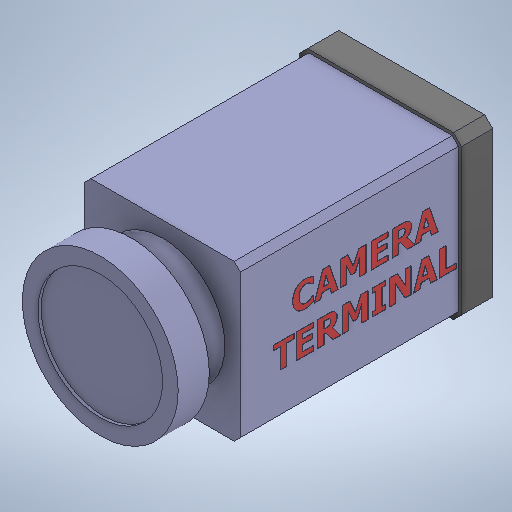
# Autodesk Inventor part: CAMERA TERMINAL
Saved by Autodesk Inventor 2025 (Build 290162000, 162)
## iProperties
Created: 2024-09-26
Part Number: CAMERA TERMINAL
Material: Generic
Document SubType Name: Modeling
Designer: DMIADX
Density: 1 g/cm^3
Appearance: Slate Blue
Author: DMIADX
Autodesk Inventor part; units mm, degrees
ref_plane "YZ Plane" through (0, 0, 0) normal (1, 0, 0) x (0, 1, 0)
ref_plane "XZ Plane" through (0, 0, 0) normal (0, 1, 0) x (-1, 0, 0)
ref_plane "XY Plane" through (0, 0, 0) normal (0, 0, 1) x (1, 0, 0)
sketch "Sketch1" plane through (0, 0, 0) normal (0, 0, 1) x (1, 0, 0)
  line L0 (25, -25) -> (-25, -25)
  line L1 (-25, -25) -> (-25, 25)
  line L2 (-25, 25) -> (25, 25)
  line L3 (25, 25) -> (25, -25)
  line L4 (25, -25) -> (-25, 25) construction
  line L5 (-25, -25) -> (25, 25) construction
  point P0 (0, 0)
  dimension "d0" = 50
  dimension "d1" = 50
  constraints: 12 end point, 2 midpoint, 2 parallel, 1 horizontal, 1 perpendicular
  measures "d0" distance of L1.end L2.end
  measures "d1" distance of L0.end L1.end
extrude "Extrusion1" add sketch "Sketch1" along normal blind 80
sketch "Sketch2" plane through (0, 0, 80) normal (0, 0, 1) x (1, 0, 0)
  circle A0 centre (0, 0) radius 25
  circle A1 centre (0, 0) radius 20
  dimension "d4" = 50
  dimension "d5" = 40
  constraints: 2 centre point, 2 coincident
  measures "d4" diameter of A0
  measures "d5" diameter of A1
extrude "Extrusion2" add sketch "Sketch2" along normal blind 19 contours A1
extrude "Extrusion3" add sketch "Sketch2" along normal blind 20
extrude "Extrusion4" cut sketch "Sketch2" along normal blind 10
sketch "Sketch3" plane through (25, -25, 0) normal (1, 0, 0) x (0, 0, -1)
  line L0 (-80, 50) -> (0, 50) construction
  line L1 (0, 50) -> (0, 0) construction
  line L2 (0, 0) -> (-80, 0) construction
  line L3 (-80, 0) -> (-80, 50) construction
  spline S0 degree 2 poles (-59.2512, 27.3525) (-61.0535, 27.3525) (-63.1669, 29.5308) (-63.1669, 31.5016) knots 0 0 0 1 2 2 2
  spline S1 degree 2 poles (-63.1669, 31.5016) (-63.1669, 33.4011) (-61.047, 35.6637) (-59.2447, 35.6637) knots 0 0 0 1 2 2 2
  spline S2 degree 2 poles (-59.2447, 35.6637) (-58.7715, 35.6637) (-58.0065, 35.5535) (-57.6564, 35.4627) knots 0 0 0 1 2 2 2
  spline S3 degree 2 poles (-57.6564, 35.4627) (-57.3841, 35.3784) (-56.7423, 35.0997) (-56.5413, 34.9959) knots 0 0 0 1 2 2 2
  line L4 (-56.5413, 34.9959) -> (-56.5413, 33.0899)
  line L5 (-56.5413, 33.0899) -> (-56.7423, 33.0899)
  spline S4 degree 2 poles (-56.7423, 33.0899) (-56.8914, 33.2196) (-57.3323, 33.5827) (-57.611, 33.7512) knots 0 0 0 1 2 2 2
  spline S5 degree 2 poles (-57.611, 33.7512) (-57.8898, 33.9263) (-58.5575, 34.1661) (-58.9271, 34.1661) knots 0 0 0 1 2 2 2
  spline S6 degree 2 poles (-58.9271, 34.1661) (-59.3614, 34.1661) (-60.081, 33.8938) (-60.4117, 33.5502) knots 0 0 0 1 2 2 2
  spline S7 degree 2 poles (-60.4117, 33.5502) (-60.7099, 33.2455) (-61.0924, 32.2018) (-61.0924, 31.4951) knots 0 0 0 1 2 2 2
  spline S8 degree 2 poles (-61.0924, 31.4951) (-61.0924, 30.7496) (-60.6969, 29.7318) (-60.3728, 29.4206) knots 0 0 0 1 2 2 2
  spline S9 degree 2 poles (-60.3728, 29.4206) (-60.0616, 29.1159) (-59.2966, 28.8501) (-58.9141, 28.8501) knots 0 0 0 1 2 2 2
  spline S10 degree 2 poles (-58.9141, 28.8501) (-58.5186, 28.8501) (-57.799, 29.1159) (-57.5527, 29.278) knots 0 0 0 1 2 2 2
  spline S11 degree 2 poles (-57.5527, 29.278) (-57.2804, 29.44) (-56.872, 29.7836) (-56.7229, 29.9198) knots 0 0 0 1 2 2 2
  line L6 (-56.7229, 29.9198) -> (-56.5413, 29.9198)
  line L7 (-56.5413, 29.9198) -> (-56.5413, 28.0397)
  spline S12 degree 2 poles (-56.5413, 28.0397) (-56.7618, 27.936) (-57.3387, 27.6767) (-57.6499, 27.5859) knots 0 0 0 1 2 2 2
  spline S13 degree 2 poles (-57.6499, 27.5859) (-58.0259, 27.4692) (-58.6807, 27.3525) (-59.2512, 27.3525) knots 0 0 0 1 2 2 2
  line L8 (-56.2172, 27.5081) -> (-53.5138, 35.5081)
  line L9 (-53.5138, 35.5081) -> (-51.3225, 35.5081)
  line L10 (-51.3225, 35.5081) -> (-48.6191, 27.5081)
  line L11 (-48.6191, 27.5081) -> (-50.6872, 27.5081)
  line L12 (-50.6872, 27.5081) -> (-51.1864, 29.1418)
  line L13 (-51.1864, 29.1418) -> (-53.7018, 29.1418)
  line L14 (-53.7018, 29.1418) -> (-54.2075, 27.5081)
  line L15 (-54.2075, 27.5081) -> (-56.2172, 27.5081)
  line L16 (-51.6272, 30.594) -> (-52.4441, 33.2391)
  line L17 (-52.4441, 33.2391) -> (-53.2674, 30.594)
  line L18 (-53.2674, 30.594) -> (-51.6272, 30.594)
  line L19 (-39.6532, 27.5081) -> (-41.6499, 27.5081)
  line L20 (-41.6499, 27.5081) -> (-41.6499, 32.8112)
  line L21 (-41.6499, 32.8112) -> (-43.1021, 29.3882)
  line L22 (-43.1021, 29.3882) -> (-44.4765, 29.3882)
  line L23 (-44.4765, 29.3882) -> (-45.9287, 32.8112)
  line L24 (-45.9287, 32.8112) -> (-45.9287, 27.5081)
  line L25 (-45.9287, 27.5081) -> (-47.8217, 27.5081)
  line L26 (-47.8217, 27.5081) -> (-47.8217, 35.5081)
  line L27 (-47.8217, 35.5081) -> (-45.5073, 35.5081)
  line L28 (-45.5073, 35.5081) -> (-43.731, 31.56)
  line L29 (-43.731, 31.56) -> (-41.9676, 35.5081)
  line L30 (-41.9676, 35.5081) -> (-39.6532, 35.5081)
  line L31 (-39.6532, 35.5081) -> (-39.6532, 27.5081)
  line L32 (-37.9935, 27.5081) -> (-37.9935, 35.5081)
  line L33 (-37.9935, 35.5081) -> (-32.5867, 35.5081)
  line L34 (-32.5867, 35.5081) -> (-32.5867, 33.9846)
  line L35 (-32.5867, 33.9846) -> (-35.9968, 33.9846)
  line L36 (-35.9968, 33.9846) -> (-35.9968, 32.5778)
  line L37 (-35.9968, 32.5778) -> (-32.8525, 32.5778)
  line L38 (-32.8525, 32.5778) -> (-32.8525, 31.0543)
  line L39 (-32.8525, 31.0543) -> (-35.9968, 31.0543)
  line L40 (-35.9968, 31.0543) -> (-35.9968, 29.0316)
  line L41 (-35.9968, 29.0316) -> (-32.5867, 29.0316)
  line L42 (-32.5867, 29.0316) -> (-32.5867, 27.5081)
  line L43 (-32.5867, 27.5081) -> (-37.9935, 27.5081)
  line L44 (-23.8347, 27.5081) -> (-26.2788, 27.5081)
  line L45 (-26.2788, 27.5081) -> (-28.5024, 30.4449)
  line L46 (-28.5024, 30.4449) -> (-29.2285, 30.4449)
  line L47 (-29.2285, 30.4449) -> (-29.2285, 27.5081)
  line L48 (-29.2285, 27.5081) -> (-31.2253, 27.5081)
  line L49 (-31.2253, 27.5081) -> (-31.2253, 35.5081)
  line L50 (-31.2253, 35.5081) -> (-28.0097, 35.5081)
  spline S14 degree 2 poles (-28.0097, 35.5081) (-27.342, 35.5081) (-26.3566, 35.3395) (-25.9352, 35.0802) knots 0 0 0 1 2 2 2
  spline S15 degree 2 poles (-25.9352, 35.0802) (-25.5073, 34.8079) (-25.0016, 33.9587) (-25.0016, 33.3104) knots 0 0 0 1 2 2 2
  spline S16 degree 2 poles (-25.0016, 33.3104) (-25.0016, 32.3963) (-25.8314, 31.2488) (-26.5251, 30.9117) knots 0 0 0 1 2 2 2
  line L51 (-26.5251, 30.9117) -> (-23.8347, 27.5081)
  spline S17 degree 2 poles (-27.0632, 33.0575) (-27.0632, 33.3622) (-27.2966, 33.7966) (-27.5624, 33.9133) knots 0 0 0 1 2 2 2
  spline S18 degree 2 poles (-27.5624, 33.9133) (-27.7504, 33.9911) (-28.2107, 34.0365) (-28.5543, 34.0365) knots 0 0 0 1 2 2 2
  line L52 (-28.5543, 34.0365) -> (-29.2285, 34.0365)
  line L53 (-29.2285, 34.0365) -> (-29.2285, 31.8841)
  line L54 (-29.2285, 31.8841) -> (-28.6515, 31.8841)
  spline S19 degree 2 poles (-28.6515, 31.8841) (-28.2366, 31.8841) (-27.6467, 31.9878) (-27.4457, 32.1499) knots 0 0 0 1 2 2 2
  spline S20 degree 2 poles (-27.4457, 32.1499) (-27.2512, 32.3055) (-27.0632, 32.7204) (-27.0632, 33.0575) knots 0 0 0 1 2 2 2
  line L55 (-24.1005, 27.5081) -> (-21.3971, 35.5081)
  line L56 (-21.3971, 35.5081) -> (-19.2058, 35.5081)
  line L57 (-19.2058, 35.5081) -> (-16.5024, 27.5081)
  line L58 (-16.5024, 27.5081) -> (-18.5705, 27.5081)
  line L59 (-18.5705, 27.5081) -> (-19.0697, 29.1418)
  line L60 (-19.0697, 29.1418) -> (-21.5851, 29.1418)
  line L61 (-21.5851, 29.1418) -> (-22.0908, 27.5081)
  line L62 (-22.0908, 27.5081) -> (-24.1005, 27.5081)
  line L63 (-19.5105, 30.594) -> (-20.3274, 33.2391)
  line L64 (-20.3274, 33.2391) -> (-21.1507, 30.594)
  line L65 (-21.1507, 30.594) -> (-19.5105, 30.594)
  line L66 (-67.1053, 14.3363) -> (-67.1053, 20.8128)
  line L67 (-67.1053, 20.8128) -> (-69.4716, 20.8128)
  line L68 (-69.4716, 20.8128) -> (-69.4716, 22.3363)
  line L69 (-69.4716, 22.3363) -> (-62.7293, 22.3363)
  line L70 (-62.7293, 22.3363) -> (-62.7293, 20.8128)
  line L71 (-62.7293, 20.8128) -> (-65.0956, 20.8128)
  line L72 (-65.0956, 20.8128) -> (-65.0956, 14.3363)
  line L73 (-65.0956, 14.3363) -> (-67.1053, 14.3363)
  line L74 (-61.906, 14.3363) -> (-61.906, 22.3363)
  line L75 (-61.906, 22.3363) -> (-56.4992, 22.3363)
  line L76 (-56.4992, 22.3363) -> (-56.4992, 20.8128)
  line L77 (-56.4992, 20.8128) -> (-59.9092, 20.8128)
  line L78 (-59.9092, 20.8128) -> (-59.9092, 19.406)
  line L79 (-59.9092, 19.406) -> (-56.765, 19.406)
  line L80 (-56.765, 19.406) -> (-56.765, 17.8825)
  line L81 (-56.765, 17.8825) -> (-59.9092, 17.8825)
  line L82 (-59.9092, 17.8825) -> (-59.9092, 15.8598)
  line L83 (-59.9092, 15.8598) -> (-56.4992, 15.8598)
  line L84 (-56.4992, 15.8598) -> (-56.4992, 14.3363)
  line L85 (-56.4992, 14.3363) -> (-61.906, 14.3363)
  line L86 (-47.7472, 14.3363) -> (-50.1912, 14.3363)
  line L87 (-50.1912, 14.3363) -> (-52.4149, 17.2731)
  line L88 (-52.4149, 17.2731) -> (-53.141, 17.2731)
  line L89 (-53.141, 17.2731) -> (-53.141, 14.3363)
  line L90 (-53.141, 14.3363) -> (-55.1378, 14.3363)
  line L91 (-55.1378, 14.3363) -> (-55.1378, 22.3363)
  line L92 (-55.1378, 22.3363) -> (-51.9222, 22.3363)
  spline S21 degree 2 poles (-51.9222, 22.3363) (-51.2545, 22.3363) (-50.269, 22.1678) (-49.8477, 21.9084) knots 0 0 0 1 2 2 2
  spline S22 degree 2 poles (-49.8477, 21.9084) (-49.4198, 21.6361) (-48.9141, 20.7869) (-48.9141, 20.1386) knots 0 0 0 1 2 2 2
  spline S23 degree 2 poles (-48.9141, 20.1386) (-48.9141, 19.2245) (-49.7439, 18.077) (-50.4376, 17.7399) knots 0 0 0 1 2 2 2
  line L93 (-50.4376, 17.7399) -> (-47.7472, 14.3363)
  spline S24 degree 2 poles (-50.9757, 19.8857) (-50.9757, 20.1904) (-51.2091, 20.6248) (-51.4749, 20.7415) knots 0 0 0 1 2 2 2
  spline S25 degree 2 poles (-51.4749, 20.7415) (-51.6629, 20.8193) (-52.1232, 20.8647) (-52.4668, 20.8647) knots 0 0 0 1 2 2 2
  line L94 (-52.4668, 20.8647) -> (-53.141, 20.8647)
  line L95 (-53.141, 20.8647) -> (-53.141, 18.7123)
  line L96 (-53.141, 18.7123) -> (-52.564, 18.7123)
  spline S26 degree 2 poles (-52.564, 18.7123) (-52.1491, 18.7123) (-51.5592, 18.8161) (-51.3582, 18.9781) knots 0 0 0 1 2 2 2
  spline S27 degree 2 poles (-51.3582, 18.9781) (-51.1637, 19.1337) (-50.9757, 19.5486) (-50.9757, 19.8857) knots 0 0 0 1 2 2 2
  line L97 (-38.9822, 14.3363) -> (-40.9789, 14.3363)
  line L98 (-40.9789, 14.3363) -> (-40.9789, 19.6394)
  line L99 (-40.9789, 19.6394) -> (-42.4311, 16.2164)
  line L100 (-42.4311, 16.2164) -> (-43.8055, 16.2164)
  line L101 (-43.8055, 16.2164) -> (-45.2577, 19.6394)
  line L102 (-45.2577, 19.6394) -> (-45.2577, 14.3363)
  line L103 (-45.2577, 14.3363) -> (-47.1507, 14.3363)
  line L104 (-47.1507, 14.3363) -> (-47.1507, 22.3363)
  line L105 (-47.1507, 22.3363) -> (-44.8363, 22.3363)
  line L106 (-44.8363, 22.3363) -> (-43.06, 18.3882)
  line L107 (-43.06, 18.3882) -> (-41.2966, 22.3363)
  line L108 (-41.2966, 22.3363) -> (-38.9822, 22.3363)
  line L109 (-38.9822, 22.3363) -> (-38.9822, 14.3363)
  line L110 (-33.342, 14.3363) -> (-37.6467, 14.3363)
  line L111 (-37.6467, 14.3363) -> (-37.6467, 15.7302)
  line L112 (-37.6467, 15.7302) -> (-36.4992, 15.7302)
  line L113 (-36.4992, 15.7302) -> (-36.4992, 20.9425)
  line L114 (-36.4992, 20.9425) -> (-37.6467, 20.9425)
  line L115 (-37.6467, 20.9425) -> (-37.6467, 22.3363)
  line L116 (-37.6467, 22.3363) -> (-33.342, 22.3363)
  line L117 (-33.342, 22.3363) -> (-33.342, 20.9425)
  line L118 (-33.342, 20.9425) -> (-34.4895, 20.9425)
  line L119 (-34.4895, 20.9425) -> (-34.4895, 15.7302)
  line L120 (-34.4895, 15.7302) -> (-33.342, 15.7302)
  line L121 (-33.342, 15.7302) -> (-33.342, 14.3363)
  line L122 (-25.154, 14.3363) -> (-27.0859, 14.3363)
  line L123 (-27.0859, 14.3363) -> (-30.1718, 19.9117)
  line L124 (-30.1718, 19.9117) -> (-30.1718, 14.3363)
  line L125 (-30.1718, 14.3363) -> (-32.0065, 14.3363)
  line L126 (-32.0065, 14.3363) -> (-32.0065, 22.3363)
  line L127 (-32.0065, 22.3363) -> (-29.543, 22.3363)
  line L128 (-29.543, 22.3363) -> (-26.9887, 17.7528)
  line L129 (-26.9887, 17.7528) -> (-26.9887, 22.3363)
  line L130 (-26.9887, 22.3363) -> (-25.154, 22.3363)
  line L131 (-25.154, 22.3363) -> (-25.154, 14.3363)
  line L132 (-24.389, 14.3363) -> (-21.6856, 22.3363)
  line L133 (-21.6856, 22.3363) -> (-19.4943, 22.3363)
  line L134 (-19.4943, 22.3363) -> (-16.7909, 14.3363)
  line L135 (-16.7909, 14.3363) -> (-18.859, 14.3363)
  line L136 (-18.859, 14.3363) -> (-19.3582, 15.97)
  line L137 (-19.3582, 15.97) -> (-21.8736, 15.97)
  line L138 (-21.8736, 15.97) -> (-22.3793, 14.3363)
  line L139 (-22.3793, 14.3363) -> (-24.389, 14.3363)
  line L140 (-19.799, 17.4222) -> (-20.6159, 20.0673)
  line L141 (-20.6159, 20.0673) -> (-21.4392, 17.4222)
  line L142 (-21.4392, 17.4222) -> (-19.799, 17.4222)
  line L143 (-10.658, 14.3363) -> (-15.9935, 14.3363)
  line L144 (-15.9935, 14.3363) -> (-15.9935, 22.3363)
  line L145 (-15.9935, 22.3363) -> (-13.9838, 22.3363)
  line L146 (-13.9838, 22.3363) -> (-13.9838, 15.8598)
  line L147 (-13.9838, 15.8598) -> (-10.658, 15.8598)
  line L148 (-10.658, 15.8598) -> (-10.658, 14.3363)
  point P0 (0, 25)
  dimension "d12" = 80
  dimension "d13" = 50
  constraints: 1 coincident, 2 other
  measures "d12" distance of L1.end L2.end
  measures "d13" distance of L0.end L1.end
sketch "Sketch4" plane through (-25, -25, 0) normal (-1, 0, 0) x (0, 0, 1)
  line L0 (0, 50) -> (80, 50) construction
  line L1 (80, 50) -> (80, 0) construction
  line L2 (80, 0) -> (0, 0) construction
  line L3 (0, 0) -> (0, 50) construction
  spline S0 degree 2 poles (20.7488, 27.3525) (18.9465, 27.3525) (16.8331, 29.5308) (16.8331, 31.5016) knots 0 0 0 1 2 2 2
  spline S1 degree 2 poles (16.8331, 31.5016) (16.8331, 33.4011) (18.953, 35.6637) (20.7553, 35.6637) knots 0 0 0 1 2 2 2
  spline S2 degree 2 poles (20.7553, 35.6637) (21.2285, 35.6637) (21.9935, 35.5535) (22.3436, 35.4627) knots 0 0 0 1 2 2 2
  spline S3 degree 2 poles (22.3436, 35.4627) (22.6159, 35.3784) (23.2577, 35.0997) (23.4587, 34.9959) knots 0 0 0 1 2 2 2
  line L4 (23.4587, 34.9959) -> (23.4587, 33.0899)
  line L5 (23.4587, 33.0899) -> (23.2577, 33.0899)
  spline S4 degree 2 poles (23.2577, 33.0899) (23.1086, 33.2196) (22.6677, 33.5827) (22.389, 33.7512) knots 0 0 0 1 2 2 2
  spline S5 degree 2 poles (22.389, 33.7512) (22.1102, 33.9263) (21.4425, 34.1661) (21.0729, 34.1661) knots 0 0 0 1 2 2 2
  spline S6 degree 2 poles (21.0729, 34.1661) (20.6386, 34.1661) (19.919, 33.8938) (19.5883, 33.5502) knots 0 0 0 1 2 2 2
  spline S7 degree 2 poles (19.5883, 33.5502) (19.2901, 33.2455) (18.9076, 32.2018) (18.9076, 31.4951) knots 0 0 0 1 2 2 2
  spline S8 degree 2 poles (18.9076, 31.4951) (18.9076, 30.7496) (19.3031, 29.7318) (19.6272, 29.4206) knots 0 0 0 1 2 2 2
  spline S9 degree 2 poles (19.6272, 29.4206) (19.9384, 29.1159) (20.7034, 28.8501) (21.0859, 28.8501) knots 0 0 0 1 2 2 2
  spline S10 degree 2 poles (21.0859, 28.8501) (21.4814, 28.8501) (22.201, 29.1159) (22.4473, 29.278) knots 0 0 0 1 2 2 2
  spline S11 degree 2 poles (22.4473, 29.278) (22.7196, 29.44) (23.128, 29.7836) (23.2771, 29.9198) knots 0 0 0 1 2 2 2
  line L6 (23.2771, 29.9198) -> (23.4587, 29.9198)
  line L7 (23.4587, 29.9198) -> (23.4587, 28.0397)
  spline S12 degree 2 poles (23.4587, 28.0397) (23.2382, 27.936) (22.6613, 27.6767) (22.3501, 27.5859) knots 0 0 0 1 2 2 2
  spline S13 degree 2 poles (22.3501, 27.5859) (21.9741, 27.4692) (21.3193, 27.3525) (20.7488, 27.3525) knots 0 0 0 1 2 2 2
  line L8 (23.7828, 27.5081) -> (26.4862, 35.5081)
  line L9 (26.4862, 35.5081) -> (28.6775, 35.5081)
  line L10 (28.6775, 35.5081) -> (31.3809, 27.5081)
  line L11 (31.3809, 27.5081) -> (29.3128, 27.5081)
  line L12 (29.3128, 27.5081) -> (28.8136, 29.1418)
  line L13 (28.8136, 29.1418) -> (26.2982, 29.1418)
  line L14 (26.2982, 29.1418) -> (25.7925, 27.5081)
  line L15 (25.7925, 27.5081) -> (23.7828, 27.5081)
  line L16 (28.3728, 30.594) -> (27.5559, 33.2391)
  line L17 (27.5559, 33.2391) -> (26.7326, 30.594)
  line L18 (26.7326, 30.594) -> (28.3728, 30.594)
  line L19 (40.3468, 27.5081) -> (38.3501, 27.5081)
  line L20 (38.3501, 27.5081) -> (38.3501, 32.8112)
  line L21 (38.3501, 32.8112) -> (36.8979, 29.3882)
  line L22 (36.8979, 29.3882) -> (35.5235, 29.3882)
  line L23 (35.5235, 29.3882) -> (34.0713, 32.8112)
  line L24 (34.0713, 32.8112) -> (34.0713, 27.5081)
  line L25 (34.0713, 27.5081) -> (32.1783, 27.5081)
  line L26 (32.1783, 27.5081) -> (32.1783, 35.5081)
  line L27 (32.1783, 35.5081) -> (34.4927, 35.5081)
  line L28 (34.4927, 35.5081) -> (36.269, 31.56)
  line L29 (36.269, 31.56) -> (38.0324, 35.5081)
  line L30 (38.0324, 35.5081) -> (40.3468, 35.5081)
  line L31 (40.3468, 35.5081) -> (40.3468, 27.5081)
  line L32 (42.0065, 27.5081) -> (42.0065, 35.5081)
  line L33 (42.0065, 35.5081) -> (47.4133, 35.5081)
  line L34 (47.4133, 35.5081) -> (47.4133, 33.9846)
  line L35 (47.4133, 33.9846) -> (44.0032, 33.9846)
  line L36 (44.0032, 33.9846) -> (44.0032, 32.5778)
  line L37 (44.0032, 32.5778) -> (47.1475, 32.5778)
  line L38 (47.1475, 32.5778) -> (47.1475, 31.0543)
  line L39 (47.1475, 31.0543) -> (44.0032, 31.0543)
  line L40 (44.0032, 31.0543) -> (44.0032, 29.0316)
  line L41 (44.0032, 29.0316) -> (47.4133, 29.0316)
  line L42 (47.4133, 29.0316) -> (47.4133, 27.5081)
  line L43 (47.4133, 27.5081) -> (42.0065, 27.5081)
  line L44 (56.1653, 27.5081) -> (53.7212, 27.5081)
  line L45 (53.7212, 27.5081) -> (51.4976, 30.4449)
  line L46 (51.4976, 30.4449) -> (50.7715, 30.4449)
  line L47 (50.7715, 30.4449) -> (50.7715, 27.5081)
  line L48 (50.7715, 27.5081) -> (48.7747, 27.5081)
  line L49 (48.7747, 27.5081) -> (48.7747, 35.5081)
  line L50 (48.7747, 35.5081) -> (51.9903, 35.5081)
  spline S14 degree 2 poles (51.9903, 35.5081) (52.658, 35.5081) (53.6434, 35.3395) (54.0648, 35.0802) knots 0 0 0 1 2 2 2
  spline S15 degree 2 poles (54.0648, 35.0802) (54.4927, 34.8079) (54.9984, 33.9587) (54.9984, 33.3104) knots 0 0 0 1 2 2 2
  spline S16 degree 2 poles (54.9984, 33.3104) (54.9984, 32.3963) (54.1686, 31.2488) (53.4749, 30.9117) knots 0 0 0 1 2 2 2
  line L51 (53.4749, 30.9117) -> (56.1653, 27.5081)
  spline S17 degree 2 poles (52.9368, 33.0575) (52.9368, 33.3622) (52.7034, 33.7966) (52.4376, 33.9133) knots 0 0 0 1 2 2 2
  spline S18 degree 2 poles (52.4376, 33.9133) (52.2496, 33.9911) (51.7893, 34.0365) (51.4457, 34.0365) knots 0 0 0 1 2 2 2
  line L52 (51.4457, 34.0365) -> (50.7715, 34.0365)
  line L53 (50.7715, 34.0365) -> (50.7715, 31.8841)
  line L54 (50.7715, 31.8841) -> (51.3485, 31.8841)
  spline S19 degree 2 poles (51.3485, 31.8841) (51.7634, 31.8841) (52.3533, 31.9878) (52.5543, 32.1499) knots 0 0 0 1 2 2 2
  spline S20 degree 2 poles (52.5543, 32.1499) (52.7488, 32.3055) (52.9368, 32.7204) (52.9368, 33.0575) knots 0 0 0 1 2 2 2
  line L55 (55.8995, 27.5081) -> (58.6029, 35.5081)
  line L56 (58.6029, 35.5081) -> (60.7942, 35.5081)
  line L57 (60.7942, 35.5081) -> (63.4976, 27.5081)
  line L58 (63.4976, 27.5081) -> (61.4295, 27.5081)
  line L59 (61.4295, 27.5081) -> (60.9303, 29.1418)
  line L60 (60.9303, 29.1418) -> (58.4149, 29.1418)
  line L61 (58.4149, 29.1418) -> (57.9092, 27.5081)
  line L62 (57.9092, 27.5081) -> (55.8995, 27.5081)
  line L63 (60.4895, 30.594) -> (59.6726, 33.2391)
  line L64 (59.6726, 33.2391) -> (58.8493, 30.594)
  line L65 (58.8493, 30.594) -> (60.4895, 30.594)
  line L66 (12.8947, 14.3363) -> (12.8947, 20.8128)
  line L67 (12.8947, 20.8128) -> (10.5284, 20.8128)
  line L68 (10.5284, 20.8128) -> (10.5284, 22.3363)
  line L69 (10.5284, 22.3363) -> (17.2707, 22.3363)
  line L70 (17.2707, 22.3363) -> (17.2707, 20.8128)
  line L71 (17.2707, 20.8128) -> (14.9044, 20.8128)
  line L72 (14.9044, 20.8128) -> (14.9044, 14.3363)
  line L73 (14.9044, 14.3363) -> (12.8947, 14.3363)
  line L74 (18.094, 14.3363) -> (18.094, 22.3363)
  line L75 (18.094, 22.3363) -> (23.5008, 22.3363)
  line L76 (23.5008, 22.3363) -> (23.5008, 20.8128)
  line L77 (23.5008, 20.8128) -> (20.0908, 20.8128)
  line L78 (20.0908, 20.8128) -> (20.0908, 19.406)
  line L79 (20.0908, 19.406) -> (23.235, 19.406)
  line L80 (23.235, 19.406) -> (23.235, 17.8825)
  line L81 (23.235, 17.8825) -> (20.0908, 17.8825)
  line L82 (20.0908, 17.8825) -> (20.0908, 15.8598)
  line L83 (20.0908, 15.8598) -> (23.5008, 15.8598)
  line L84 (23.5008, 15.8598) -> (23.5008, 14.3363)
  line L85 (23.5008, 14.3363) -> (18.094, 14.3363)
  line L86 (32.2528, 14.3363) -> (29.8088, 14.3363)
  line L87 (29.8088, 14.3363) -> (27.5851, 17.2731)
  line L88 (27.5851, 17.2731) -> (26.859, 17.2731)
  line L89 (26.859, 17.2731) -> (26.859, 14.3363)
  line L90 (26.859, 14.3363) -> (24.8622, 14.3363)
  line L91 (24.8622, 14.3363) -> (24.8622, 22.3363)
  line L92 (24.8622, 22.3363) -> (28.0778, 22.3363)
  spline S21 degree 2 poles (28.0778, 22.3363) (28.7455, 22.3363) (29.731, 22.1678) (30.1523, 21.9084) knots 0 0 0 1 2 2 2
  spline S22 degree 2 poles (30.1523, 21.9084) (30.5802, 21.6361) (31.0859, 20.7869) (31.0859, 20.1386) knots 0 0 0 1 2 2 2
  spline S23 degree 2 poles (31.0859, 20.1386) (31.0859, 19.2245) (30.2561, 18.077) (29.5624, 17.7399) knots 0 0 0 1 2 2 2
  line L93 (29.5624, 17.7399) -> (32.2528, 14.3363)
  spline S24 degree 2 poles (29.0243, 19.8857) (29.0243, 20.1904) (28.7909, 20.6248) (28.5251, 20.7415) knots 0 0 0 1 2 2 2
  spline S25 degree 2 poles (28.5251, 20.7415) (28.3371, 20.8193) (27.8768, 20.8647) (27.5332, 20.8647) knots 0 0 0 1 2 2 2
  line L94 (27.5332, 20.8647) -> (26.859, 20.8647)
  line L95 (26.859, 20.8647) -> (26.859, 18.7123)
  line L96 (26.859, 18.7123) -> (27.436, 18.7123)
  spline S26 degree 2 poles (27.436, 18.7123) (27.8509, 18.7123) (28.4408, 18.8161) (28.6418, 18.9781) knots 0 0 0 1 2 2 2
  spline S27 degree 2 poles (28.6418, 18.9781) (28.8363, 19.1337) (29.0243, 19.5486) (29.0243, 19.8857) knots 0 0 0 1 2 2 2
  line L97 (41.0178, 14.3363) -> (39.0211, 14.3363)
  line L98 (39.0211, 14.3363) -> (39.0211, 19.6394)
  line L99 (39.0211, 19.6394) -> (37.5689, 16.2164)
  line L100 (37.5689, 16.2164) -> (36.1945, 16.2164)
  line L101 (36.1945, 16.2164) -> (34.7423, 19.6394)
  line L102 (34.7423, 19.6394) -> (34.7423, 14.3363)
  line L103 (34.7423, 14.3363) -> (32.8493, 14.3363)
  line L104 (32.8493, 14.3363) -> (32.8493, 22.3363)
  line L105 (32.8493, 22.3363) -> (35.1637, 22.3363)
  line L106 (35.1637, 22.3363) -> (36.94, 18.3882)
  line L107 (36.94, 18.3882) -> (38.7034, 22.3363)
  line L108 (38.7034, 22.3363) -> (41.0178, 22.3363)
  line L109 (41.0178, 22.3363) -> (41.0178, 14.3363)
  line L110 (46.658, 14.3363) -> (42.3533, 14.3363)
  line L111 (42.3533, 14.3363) -> (42.3533, 15.7302)
  line L112 (42.3533, 15.7302) -> (43.5008, 15.7302)
  line L113 (43.5008, 15.7302) -> (43.5008, 20.9425)
  line L114 (43.5008, 20.9425) -> (42.3533, 20.9425)
  line L115 (42.3533, 20.9425) -> (42.3533, 22.3363)
  line L116 (42.3533, 22.3363) -> (46.658, 22.3363)
  line L117 (46.658, 22.3363) -> (46.658, 20.9425)
  line L118 (46.658, 20.9425) -> (45.5105, 20.9425)
  line L119 (45.5105, 20.9425) -> (45.5105, 15.7302)
  line L120 (45.5105, 15.7302) -> (46.658, 15.7302)
  line L121 (46.658, 15.7302) -> (46.658, 14.3363)
  line L122 (54.846, 14.3363) -> (52.9141, 14.3363)
  line L123 (52.9141, 14.3363) -> (49.8282, 19.9117)
  line L124 (49.8282, 19.9117) -> (49.8282, 14.3363)
  line L125 (49.8282, 14.3363) -> (47.9935, 14.3363)
  line L126 (47.9935, 14.3363) -> (47.9935, 22.3363)
  line L127 (47.9935, 22.3363) -> (50.457, 22.3363)
  line L128 (50.457, 22.3363) -> (53.0113, 17.7528)
  line L129 (53.0113, 17.7528) -> (53.0113, 22.3363)
  line L130 (53.0113, 22.3363) -> (54.846, 22.3363)
  line L131 (54.846, 22.3363) -> (54.846, 14.3363)
  line L132 (55.611, 14.3363) -> (58.3144, 22.3363)
  line L133 (58.3144, 22.3363) -> (60.5057, 22.3363)
  line L134 (60.5057, 22.3363) -> (63.2091, 14.3363)
  line L135 (63.2091, 14.3363) -> (61.141, 14.3363)
  line L136 (61.141, 14.3363) -> (60.6418, 15.97)
  line L137 (60.6418, 15.97) -> (58.1264, 15.97)
  line L138 (58.1264, 15.97) -> (57.6207, 14.3363)
  line L139 (57.6207, 14.3363) -> (55.611, 14.3363)
  line L140 (60.201, 17.4222) -> (59.3841, 20.0673)
  line L141 (59.3841, 20.0673) -> (58.5608, 17.4222)
  line L142 (58.5608, 17.4222) -> (60.201, 17.4222)
  line L143 (69.342, 14.3363) -> (64.0065, 14.3363)
  line L144 (64.0065, 14.3363) -> (64.0065, 22.3363)
  line L145 (64.0065, 22.3363) -> (66.0162, 22.3363)
  line L146 (66.0162, 22.3363) -> (66.0162, 15.8598)
  line L147 (66.0162, 15.8598) -> (69.342, 15.8598)
  line L148 (69.342, 15.8598) -> (69.342, 14.3363)
  point P0 (0, 25)
  point P1 (64.7728, 17.8317)
  dimension "d14" = 80
  dimension "d15" = 50
  constraints: 2 coincident, 2 other
  measures "d14" distance of L1.end L2.end
  measures "d15" distance of L0.end L1.end
emboss "Emboss1" sketch "Sketch4" operation cut depth 0.1 direction (1, 0, 0)
emboss "Emboss2" sketch "Sketch3" operation cut depth 0.1 direction (-1, 0, 0)
chamfer "Chamfer1" distance 2 angle 45 4 edges at (-25, 25, 40) (25, 25, 40) (25, -25, 40) (-25, -25, 40)
sketch "Sketch5" plane through (0, 0, 0) normal (0, 0, -1) x (-1, 0, 0)
  line L0 (25, -23) -> (23, -25) projected
  line L1 (25, 23) -> (25, -23) projected
  line L2 (23, 25) -> (25, 23) projected
  line L3 (-23, 25) -> (23, 25) projected
  line L4 (-25, 23) -> (-23, 25) projected
  line L5 (-25, -23) -> (-25, 23) projected
  line L6 (-23, -25) -> (-25, -23) projected
  line L7 (23, -25) -> (-23, -25) projected
  line L8 (26, -23.4142) -> (23.4142, -26)
  line L9 (23.4142, -26) -> (-23.4142, -26)
  line L10 (-23.4142, -26) -> (-26, -23.4142)
  line L11 (-26, -23.4142) -> (-26, 23.4142)
  line L12 (-26, 23.4142) -> (-23.4142, 26)
  line L13 (-23.4142, 26) -> (23.4142, 26)
  line L14 (23.4142, 26) -> (26, 23.4142)
  line L15 (26, 23.4142) -> (26, -23.4142)
  point P0 (0, 0)
  dimension "d23" = 1
  constraints: 16 end point, 7 other
  measures "d23" distance between parallel lines of L1 L15
extrude "Extrusion5" add sketch "Sketch5" against normal blind 10 contours L0 L7 L6 L5 L4 L3 L2 L1 | L8 L9 L10 L11 L12 L13 L14 L15
body "Solid1"
